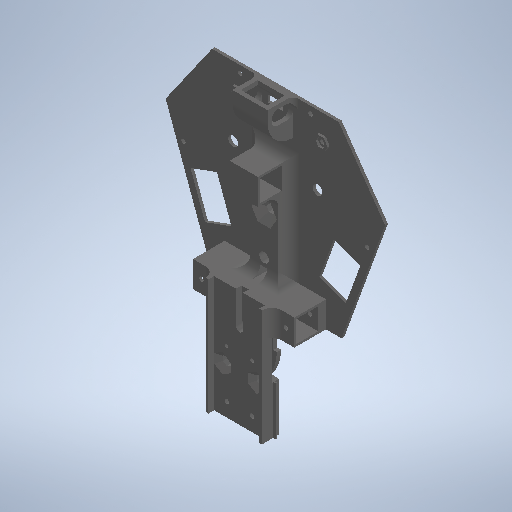
# Autodesk Inventor part: back_board_setter
Saved by Autodesk Inventor 2026.1 (Build 301233020, 233B)
## iProperties
Created: 2026-02-04
Part Number: back_board_setter
Material: 一般
Document SubType Name: Modeling
Designer: hibik
Density: 1 g/cm^3
Appearance: 既定
Author: hibik
Autodesk Inventor part; units mm, degrees
ref_plane "YZ Plane" through (0, 0, 0) normal (1, 0, 0) x (0, 1, 0)
ref_plane "XY Plane" through (0, 0, 0) normal (0, 0, 1) x (1, 0, 0)
sketch "スケッチ1" plane through (0, 0, 0) normal (0, 0, 1) x (1, 0, 0)
  line L0 (-36, -9.25) -> (36, -9.25)
  line L1 (36, -9.25) -> (36, 9.25)
  line L2 (36, 9.25) -> (-36, 9.25)
  line L3 (-36, 9.25) -> (-36, -9.25)
  point P0 (0, 0)
  point P1 (0, 9.25)
  point P2 (-36, 0)
  dimension "d0" = 72
  dimension "d1" = 18.5
  constraints: 8 end point, 2 midpoint, 2 parallel, 1 horizontal, 1 horizontal alignment, 1 perpendicular, 1 vertical alignment
  measures "d0" distance of L2.end L1.end
  measures "d1" distance of L2.end L0.start
extrude "押し出し1" add sketch "スケッチ1" along normal mid plane 18.5
shell "シェル1" thickness 1.5 removed faces 2 at (36, 3.0833, 3.0833) at (-36, 3.0833, -3.0833)
sketch "スケッチ2" plane through (0, 0, 9.25) normal (0, 0, 1) x (1, 0, 0)
  circle A0 centre (-30, 0) radius 1.6
  line L0 (0, -12.95) -> (0, 12.95) projected
  circle A1 centre (30, 0) radius 1.6
  line L1 (-36, 9.25) -> (-36, -9.25) projected
  point P0 (0, 0)
  dimension "d5" = 3.2
  dimension "d6" = 6
  constraints: 2 centre point, 1 horizontal alignment, 1 other
  measures "d5" diameter of A0
  measures "d6" distance from line of L1 A0.centre
extrude "押し出し2" cut sketch "スケッチ2" against normal through all
sketch "スケッチ3" plane through (0, 0, -9.25) normal (0, 0, -1) x (-1, 0, 0)
  line L0 (-10, 64.25) -> (10, 64.25)
  line L1 (10, 64.25) -> (10, -9.25)
  line L2 (10, -9.25) -> (-10, -9.25)
  line L3 (-10, -9.25) -> (-10, 64.25)
  line L4 (-36, -9.25) -> (36, -9.25) projected
  line L5 (-36, 9.25) -> (36, 9.25) projected
  line L6 (-10, 9.25) -> (10, 9.25)
  point P0 (0, 0)
  point P1 (0, -9.25)
  dimension "d14" = 64.25
  dimension "d15" = 20
  constraints: 10 end point, 4 point on line, 2 parallel, 1 collinear, 1 horizontal, 1 midpoint, 1 perpendicular, 1 vertical alignment
  measures "d14" distance from line of L0 point (0, 0)
  measures "d15" distance of L0.start L0.end
extrude "押し出し3" add sketch "スケッチ3" along normal mid plane 8 contours L0 L1 L5 L3
ref_plane "作業平面1" through (0, 73.5, 0) normal (0, 1, 0) x (-1, 0, 0)
sketch "スケッチ4" plane through (0, 0, 0) normal (1, 0, 0) x (0, 1, 0)
  line L0 (73.5, 14.95) -> (73.5, -24.95) projected
  line L1 (81.25, 7.75) -> (65.75, 7.75)
  line L2 (65.75, 7.75) -> (65.75, -7.75)
  line L3 (65.75, -7.75) -> (81.25, -7.75)
  line L4 (81.25, -7.75) -> (81.25, 7.75)
  line L5 (81.25, 7.75) -> (65.75, -7.75) construction
  line L6 (65.75, 7.75) -> (81.25, -7.75) construction
  line L7 (7.75, -7.75) -> (-7.75, -7.75) projected
  line L8 (82.75, 9.25) -> (64.25, 9.25)
  line L9 (64.25, 9.25) -> (64.25, -9.25)
  line L10 (64.25, -9.25) -> (82.75, -9.25)
  line L11 (82.75, -9.25) -> (82.75, 9.25)
  line L12 (82.75, 9.25) -> (64.25, -9.25) construction
  line L13 (64.25, 9.25) -> (82.75, -9.25) construction
  line L14 (-9.25, 9.25) -> (9.25, 9.25) projected
  point P0 (0, 0)
  point P1 (73.5, 0)
  constraints: 24 end point, 4 equal length, 4 midpoint, 4 parallel, 2 horizontal, 2 perpendicular, 1 horizontal alignment, 1 point on line
extrude "押し出し4" add sketch "スケッチ4" along normal mid plane 20 contours L8 L11 L10 L0 L3 L4 L1 | L0 L1 L2 L3 L10 L9 L8
sketch "スケッチ7" plane through (0, 0, 9.25) normal (0, 0, 1) x (1, 0, 0)
  line L0 (-36, 9.25) -> (-10, 9.25) projected
  line L1 (-20, 9.25) -> (20, 9.25)
  line L2 (20, 9.25) -> (20, -73.25)
  line L3 (20, -73.25) -> (-20, -73.25)
  line L4 (-20, -73.25) -> (-20, 9.25)
  line L5 (-36, -9.25) -> (36, -9.25) projected
  point P0 (0, 0)
  point P1 (0, -73.25)
  point P2 (-10, 9.25)
  dimension "d27" = 40
  dimension "d28" = 64
  constraints: 8 end point, 2 parallel, 1 horizontal, 1 midpoint, 1 perpendicular, 1 point on line, 1 vertical alignment
  measures "d27" distance of L2.end L3.end
  measures "d28" distance between parallel lines of L3 L5
extrude "押し出し7" add sketch "スケッチ7" along normal blind 7
sketch "スケッチ8" plane through (0, 0, 16.25) normal (0, 0, 1) x (1, 0, 0)
  line L0 (10, 9.25) -> (36, 9.25) projected
  line L1 (-18, -73.25) -> (18, -73.25)
  line L2 (18, -73.25) -> (18, 9.25)
  line L3 (18, 9.25) -> (-18, 9.25)
  line L4 (-18, 9.25) -> (-18, -73.25)
  line L5 (-20, -73.25) -> (20, -73.25) projected
  line L6 (-20, 9.25) -> (-20, -73.25) projected
  point P0 (0, 0)
  point P1 (0, -73.25)
  dimension "d31" = 2
  constraints: 8 end point, 2 midpoint, 2 parallel, 2 point on line, 1 horizontal, 1 perpendicular
  measures "d31" distance between parallel lines of L6 L4
extrude "押し出し8" cut sketch "スケッチ8" against normal blind 4
sketch "スケッチ9" plane through (0, 0, 9.25) normal (0, 0, -1) x (-1, 0, 0)
  line L0 (20, -9.25) -> (-20, -9.25) projected
  line L1 (-20, -73.25) -> (-20, -9.25) projected
  line L2 (20, -73.25) -> (-20, -73.25) projected
  line L3 (20, -9.25) -> (20, -73.25) projected
  point P0 (0, 0)
extrude "押し出し9" add sketch "スケッチ9" along normal blind 5
sketch "スケッチ10" plane through (0, 0, 4.25) normal (0, 0, -1) x (-1, 0, 0)
  circle A0 centre (-12, -41.25) radius 1.6
  line L0 (0, -104.45) -> (0, 113.95) projected
  circle A1 centre (12, -41.25) radius 1.6
  line L1 (-20, -9.25) -> (-20, -73.25) projected
  point P0 (0, 0)
  point P1 (-20, -41.25)
  dimension "d36" = 3.2
  dimension "d37" = 24
  constraints: 2 centre point, 1 horizontal alignment, 1 midpoint, 1 other
  measures "d36" diameter of A0
  measures "d37" distance of A1.centre A0.centre
extrude "押し出し10" cut sketch "スケッチ10" against normal through all
sketch "スケッチ11" plane through (0, 0, -13.25) normal (0, 0, -1) x (-1, 0, 0)
  line L0 (-72.5487, 98.7272) -> (-55.0126, 50.5473) projected
  line L1 (72.5487, 98.7272) -> (55.0126, 50.5473) projected
  line L2 (-95, 122.75) -> (95, 122.75)
  line L3 (95, 122.75) -> (46.9559, -9.25)
  line L4 (46.9559, -9.25) -> (-46.9559, -9.25)
  line L5 (-46.9559, -9.25) -> (-95, 122.75)
  line L6 (0, -107.6454) -> (0, 133.1226) projected
  line L7 (10, 82.75) -> (-10, 82.75) projected
  line L8 (-36, -9.25) -> (36, -9.25) projected
  point P0 (0, 0)
  dimension "d40" = 190
  dimension "d56" = 40
  constraints: 8 end point, 2 parallel, 1 collinear, 1 horizontal, 1 other
  measures "d40" distance of L2.start L2.end
  measures "d56" distance between parallel lines of L2 L7
extrude "押し出し11" add sketch "スケッチ11" along normal blind 2
sketch "スケッチ12" plane through (10, 82.75, -9.25) normal (0, 0, -1) x (-1, 0, 0)
  line L0 (20, 0) -> (0, 0) projected
  line L1 (0, -18.5) -> (0, 0) projected
  line L2 (20, -18.5) -> (0, -18.5) projected
  line L3 (20, 0) -> (20, -18.5) projected
  point P0 (10, -82.75)
extrude "押し出し12" add sketch "スケッチ12" along normal up to surface (4 mm away)
sketch "スケッチ13" plane through (0, 0, -9.25) normal (0, 0, -1) x (-1, 0, 0)
  circle A0 centre (-30, 0) radius 1.6 projected
  circle A1 centre (30, 0) radius 1.6 projected
  circle A2 centre (-30, 0) radius 3.5
  circle A3 centre (30, 0) radius 3.5
  circle A4 centre (30, 73.5) radius 1.6 projected
  circle A5 centre (-30, 73.5) radius 1.6 projected
  circle A6 centre (-30, 73.5) radius 3.5
  circle A7 centre (30, 73.5) radius 3.5
  point P0 (0, 0)
  dimension "d45" = 7
  dimension "d46" = 7
  dimension "d47" = 7
  dimension "d48" = 7
  constraints: 4 centre point, 4 coincident
  measures "d45" diameter of A2
  measures "d46" diameter of A3
  measures "d47" diameter of A6
  measures "d48" diameter of A7
extrude "押し出し13" cut sketch "スケッチ13" along normal through all contours A0 | A1 | A2 | A3 | A4 | A5 | A6 | A7
sketch "スケッチ14" plane through (0, 0, -15.25) normal (0, 0, -1) x (-1, 0, 0)
  circle A0 centre (30, 0) radius 3.5 projected
  line L0 (46.9559, -9.25) -> (95, 122.75) projected
  line L1 (95, 122.75) -> (-95, 122.75) projected
  line L2 (-95, 122.75) -> (-46.9559, -9.25) projected
  circle A1 centre (-30, 0) radius 3.5 projected
  line L3 (-46.9559, -9.25) -> (46.9559, -9.25) projected
  circle A2 centre (30, 73.5) radius 3.5 projected
  circle A3 centre (-30, 73.5) radius 3.5 projected
  circle A4 centre (30, 0) radius 1.6 projected
  circle A5 centre (-30, 0) radius 1.6 projected
  line L4 (-36, 9.25) -> (-36, -9.25) projected
  line L5 (-36, -9.25) -> (36, -9.25) projected
  line L6 (36, -9.25) -> (36, 9.25) projected
  line L7 (36, 9.25) -> (10, 9.25) projected
  line L8 (10, 9.25) -> (-10, 9.25) projected
  line L9 (-10, 9.25) -> (-36, 9.25) projected
  point P0 (0, 0)
  point P1 (33.2482, 9.25)
  point P2 (-33.2482, 9.25)
extrude "押し出し14" add sketch "スケッチ14" against normal up to surface (6 mm away) contours L3 L4 L9 L8 L7 L6
chamfer "面取り1" distance 50 angle 45 2 edges at (-95, 122.75, -14.25) (95, 122.75, -14.25)
fillet "フィレット3" radius 7 11 edges at (-10, 46, -13.25) (0, 82.75, -13.25) (10, 46, -13.25) (0, 9.25, -5.25) (-10, 9.25, -7.25) (-10, 9.25, -11.25) (10, 9.25, -11.25) (10, 9.25, -7.25) (-20, 0, 9.25) (20, 0, 9.25) (0, 64.25, -5.25)
sketch "スケッチ16" plane through (0, 0, -13.25) normal (0, 0, 1) x (1, 0, 0)
  line L0 (-60.2509, 41.8965) -> (-49.9903, 13.7058)
  line L1 (-49.9903, 13.7058) -> (-31.1964, 20.5462)
  line L2 (-31.1964, 20.5462) -> (-41.457, 48.7369)
  line L3 (-41.457, 48.7369) -> (-60.2509, 41.8965)
  line L4 (-46.9559, -9.25) -> (-77.899, 75.7654) projected
  point P0 (0, 0)
  point P1 (-43, 16.25)
  dimension "d66" = 5
  dimension "d67" = 20
  dimension "d68" = 30
  constraints: 8 end point, 3 parallel, 1 perpendicular, 1 point on line
  measures "d66" distance between parallel lines of L4 L0
  measures "d67" distance between parallel lines of L0 L2
  measures "d68" distance between parallel lines of L1 L3
extrude "押し出し16" cut sketch "スケッチ16" against normal through all
sketch "スケッチ17" plane through (0, 0, -13.25) normal (0, 0, 1) x (1, 0, 0)
  circle A0 centre (-65.2987, 55.7654) radius 1.6
  circle A1 centre (-65.2987, 55.7654) radius 5
  circle A2 centre (-25, 117.75) radius 5
  circle A3 centre (-25, 117.75) radius 1.6
  circle A4 centre (0, 21) radius 5
  circle A5 centre (0, 21) radius 1.6
  line L0 (-46.9559, -9.25) -> (-77.899, 75.7654) projected
  line L1 (-45, 122.75) -> (45, 122.75) projected
  point P0 (0, 0)
  dimension "d71" = 3.2
  dimension "d72" = 10
  dimension "d74" = 21
  dimension "d75" = 25
  dimension "d76" = 20
  constraints: 6 centre point, 4 equal radius, 3 coincident, 2 tangent, 1 vertical alignment
  measures "d71" diameter of A0
  measures "d72" diameter of A1
  measures "d74" distance of point (0, 0) A4.centre
  measures "d75" horizontal distance of point (0, 0) A2.centre
  measures "d76" vertical distance of L0.end A0.centre
extrude "押し出し17" cut sketch "スケッチ17" along normal mid plane 100 contours A0 | A3 | A5
sketch "スケッチ18" plane through (0, 0, -5.25) normal (0, 0, 1) x (1, 0, 0)
  circle A0 centre (0, 21) radius 1.6 projected
  circle A1 centre (0, 21) radius 3.5
  point P0 (0, 0)
  dimension "d79" = 7
  constraints: 1 centre point, 1 coincident
  measures "d79" diameter of A1
extrude "押し出し18" cut sketch "スケッチ18" against normal up to surface (8 mm away) contours A0 | A1
mirror "ミラー1" about plane through (0, 0, 0) normal (1, 0, 0) of "押し出し17", "押し出し16"
sketch "スケッチ19" plane through (-20, -9.25, 4.25) normal (0, -1, 0) x (1, 0, 0)
  line L0 (40, 12) -> (40, 0) projected
  line L1 (0, 0) -> (0, 12) projected
  line L2 (42, 3) -> (-2, 3)
  line L3 (-2, 3) -> (-2, 4)
  line L4 (-2, 4) -> (42, 4)
  line L5 (42, 4) -> (42, 3)
  line L6 (40, 0) -> (0, 0) projected
  point P0 (20, -4.25)
  point P1 (20, 0)
  point P2 (20, 3)
  point P3 (40, 4)
  point P4 (40, 3)
  point P5 (0, 3)
  point P6 (0, 4)
  dimension "d82" = 2
  dimension "d83" = 3
  dimension "d84" = 1
  constraints: 8 end point, 2 midpoint, 2 parallel, 1 horizontal, 1 perpendicular, 1 vertical alignment
  measures "d82" distance between parallel lines of L0 L5
  measures "d83" distance between parallel lines of L6 L2
  measures "d84" distance of L4.end L2.start
extrude "押し出し19" add sketch "スケッチ19" along normal up to surface (64 mm away) contours L4 L5 L2 L0 | L1 L2 L3 L4
sketch "スケッチ20" plane through (-45, 122.75, -13.25) normal (0, 1, 0) x (1, 0, 0)
  line L0 (54.5, -3) -> (35.5, -3)
  line L1 (35.5, -3) -> (35.5, -15)
  line L2 (35.5, -15) -> (54.5, -15)
  line L3 (54.5, -15) -> (54.5, -3)
  line L4 (57.5, 0) -> (32.5, 0)
  line L5 (32.5, 0) -> (32.5, -18)
  line L6 (32.5, -18) -> (57.5, -18)
  line L7 (57.5, -18) -> (57.5, 0)
  line L8 (0, 0) -> (90, 0) projected
  point P0 (45, -13.25)
  point P1 (54.5, -9)
  point P2 (57.5, -9)
  point P3 (45, 0)
  point P4 (45, 0)
  point P5 (45, -3)
  point P6 (45, 0)
  dimension "d87" = 19
  dimension "d88" = 12
  dimension "d89" = 3
  dimension "d90" = 3
  constraints: 16 end point, 6 midpoint, 4 parallel, 2 horizontal, 2 perpendicular, 1 coincident, 1 horizontal alignment, 1 point on line, 1 vertical alignment
  measures "d87" distance of L2.end L1.end
  measures "d88" distance of L1.end L0.end
  measures "d89" distance between parallel lines of L7 L3
  measures "d90" distance between parallel lines of L6 L2
extrude "押し出し20" add sketch "スケッチ20" against normal blind 3
sketch "スケッチ21" plane through (-12.5, 122.75, -13.25) normal (-1, 0, 0) x (0, 0, 1)
  line L0 (18, 0) -> (18, -3) projected
  line L1 (15, -3) -> (18, -3)
  line L2 (18, -3) -> (18, -8)
  line L3 (18, -8) -> (15, -8)
  line L4 (15, -8) -> (15, -3)
  arc A0 (0, -23) -> (15, -8) centre (0, -8) ccw
  arc A1 (0, -26) -> (18, -8) centre (0, -8) ccw
  line L5 (0, -3.4) -> (0, -6.6) projected
  line L6 (0, -65.3846) -> (0, -68.5846) projected
  line L7 (0, -65.3846) -> (0, -68.5846) projected
  line L8 (0, -3.4) -> (0, -6.6) projected
  line L9 (0, -45.75) -> (0, -52.75) projected
  line L10 (0, -45.75) -> (0, -52.75) projected
  line L11 (0, 0) -> (0, -3) projected
  line L12 (0, -3) -> (0, 0) projected
  line L13 (0, -46.9846) -> (0, 0) projected
  line L14 (0, -132) -> (0, -46.9846) projected
  line L15 (0, -102.2038) -> (0, -109.0442) projected
  line L16 (0, -109.0442) -> (0, -80.8535) projected
  line L17 (0, -80.8535) -> (0, -74.0131) projected
  line L18 (0, -74.0131) -> (0, -102.2038) projected
  line L19 (0, -33) -> (0, -113.5) projected
  line L20 (0, -113.5) -> (0, -33) projected
  line L21 (0, -109.0442) -> (0, -102.2038) projected
  line L22 (0, -102.2038) -> (0, -74.0131) projected
  line L23 (0, -74.0131) -> (0, -80.8535) projected
  line L24 (0, -80.8535) -> (0, -109.0442) projected
  line L25 (0, -46.9846) -> (0, -132) projected
  line L26 (0, 0) -> (0, -46.9846) projected
  line L27 (0, -23) -> (7.534, -23)
  line L28 (0, -132) -> (0, -113.5) projected
  line L29 (0, -113.5) -> (0, -132) projected
  point P0 (13.25, -122.75)
  point P1 (15, 0)
  point P2 (0, -23)
  dimension "d93" = 5
  constraints: 10 end point, 4 point on circle, 2 centre point, 2 horizontal, 2 parallel, 2 point on line, 2 tangent, 1 collinear, 1 concentric, 1 perpendicular
  measures "d93" distance of L1.end L2.end
extrude "押し出し21" add sketch "スケッチ21" against normal up to surface (25 mm away)
sketch "スケッチ22" plane through (0, 0, 4.25) normal (0, 0, -1) x (-1, 0, 0)
  line L0 (20, -9.25) -> (20, -73.25) projected
  line L1 (20, -19.25) -> (22.5, -19.25)
  arc A0 (16, -37.25) -> (22.5, -19.25) centre (-5.6731, -19.25) ccw
  line L2 (22.5, -19.25) -> (22.5, -28.0637)
  line L3 (16, -37.25) -> (16, -9.25)
  line L4 (16, -9.25) -> (20, -9.25)
  line L5 (-20, -9.25) -> (20, -9.25) projected
  line L6 (11.6828, -9.25) -> (37.771, -9.25)
  line L7 (37.771, -9.25) -> (37.771, -40.25)
  line L8 (37.771, -40.25) -> (11.6828, -40.25)
  line L9 (11.6828, -40.25) -> (11.6828, -9.25)
  circle A1 centre (20, -9.25) radius 29.6886
  point P0 (0, 0)
  point P1 (11.6828, -37.7498)
  point P2 (37.771, -33.0325)
  dimension "d96" = 4
  dimension "d97" = 2.5
  dimension "d98" = 10
  dimension "d99" = 18
  dimension "d100" = 3
  constraints: 16 end point, 3 perpendicular, 2 centre point, 2 horizontal, 2 parallel, 2 point on circle, 2 point on line, 1 coincident, 1 tangent, 1 vertical
  measures "d96" distance between parallel lines of L0 L3
  measures "d97" distance of L1.start L1.end
  measures "d98" distance from line of L1.start L4
  measures "d99" vertical distance of L1.end L3.start
  measures "d100" distance from line of L8 L3.start
extrude "押し出し22" cut sketch "スケッチ22" against normal blind 5 contours L6 L7 A1 L0 A0 L1 | L0 A0 L3 L4 | L1 A0 L0 | L3 A0 L0 A1 L9 L5
extrude "押し出し23" add sketch "スケッチ22" against normal blind 4 contours L0 A0 L3 L4 | L1 A0 L0
extrude "押し出し24" cut sketch "スケッチ22" against normal blind 1 contours L0 A0 L3 L4 | L1 A0 L0
mirror "ミラー2" about plane through (0, 0, 0) normal (1, 0, 0) of "押し出し22", "押し出し23", "押し出し24"
sketch "スケッチ23" plane through (0, 0, 12.25) normal (0, 0, 1) x (1, 0, 0)
  circle A0 centre (-9, -63.25) radius 1.3
  circle A1 centre (9, -63.25) radius 1.3
  line L0 (18, -73.25) -> (-18, -73.25) projected
  line L1 (0, -73.25) -> (0, 0)
  circle A2 centre (-9, -29.25) radius 1.3
  circle A3 centre (9, -29.25) radius 1.3
  dimension "d107" = 2.6
  dimension "d109" = 18
  dimension "d112" = 34
  dimension "d117" = 10
  constraints: 4 centre point, 2 end point, 2 vertical, 1 midpoint, 5 other
  measures "d107" diameter of A0
  measures "d109" distance of A1.centre A0.centre
  measures "d112" distance of A0.centre A2.centre
  measures "d117" distance from line of L0 A0.centre
extrude "押し出し25" cut sketch "スケッチ23" against normal up to surface (3 mm away)
sketch "スケッチ24" plane through (0, 0, 12.25) normal (0, 0, 1) x (1, 0, 0)
  circle A0 centre (-9, -63.25) radius 1.3 projected
  circle A1 centre (9, -63.25) radius 1.3 projected
  circle A2 centre (-9, -63.25) radius 1.6
  circle A3 centre (9, -63.25) radius 1.6
  point P0 (0, 0)
  dimension "d120" = 3.2
  dimension "d121" = 3.2
  constraints: 2 centre point, 2 coincident
  measures "d120" diameter of A2
  measures "d121" diameter of A3
extrude "押し出し26" cut sketch "スケッチ24" against normal through all contours A0 | A1 | A2 | A3
sketch "スケッチ25" plane through (0, 0, 4.25) normal (0, 0, -1) x (-1, 0, 0)
  circle A0 centre (-9, -63.25) radius 1.6 projected
  line L0 (-7.3546, -66.1) -> (-10.6454, -66.1)
  line L1 (-10.6454, -66.1) -> (-12.2909, -63.25)
  line L2 (-12.2909, -63.25) -> (-10.6454, -60.4)
  line L3 (-10.6454, -60.4) -> (-7.3546, -60.4)
  line L4 (-7.3546, -60.4) -> (-5.7091, -63.25)
  line L5 (-5.7091, -63.25) -> (-7.3546, -66.1)
  circle A1 centre (9, -63.25) radius 1.6 projected
  line L6 (7.3546, -66.1) -> (5.7091, -63.25)
  line L7 (5.7091, -63.25) -> (7.3546, -60.4)
  line L8 (7.3546, -60.4) -> (10.6454, -60.4)
  line L9 (10.6454, -60.4) -> (12.2909, -63.25)
  line L10 (12.2909, -63.25) -> (10.6454, -66.1)
  line L11 (10.6454, -66.1) -> (7.3546, -66.1)
  point P0 (0, 0)
  dimension "d124" = 5.7
  constraints: 24 end point, 2 coincident, 1 collinear, 1 horizontal, 1 horizontal alignment, 26 other
  measures "d124" distance between parallel lines of L0 L3
extrude "押し出し27" cut sketch "スケッチ25" against normal blind 6 contours A0 | L0 L1 L2 L3 L4 L5 | A1 | L6 L7 L8 L9 L10 L11
chamfer "面取り2" distance 4 angle 45 12 edges at (9, -60.4, 4.25) (6.5318, -61.825, 4.25) (6.5318, -64.675, 4.25) (9, -66.1, 4.25) (11.4682, -64.675, 4.25) (11.4682, -61.825, 4.25) (-6.5318, -61.825, 4.25) (-6.5318, -64.675, 4.25) (-9, -66.1, 4.25) (-11.4682, -64.675, 4.25) (-11.4682, -61.825, 4.25) (-9, -60.4, 4.25)
sketch "スケッチ26" plane through (0, 0, 12.25) normal (0, 0, 1) x (1, 0, 0)
  circle A0 centre (-12, -41.25) radius 1.6 projected
  circle A1 centre (12, -41.25) radius 1.6 projected
  line L0 (-9.15, -42.8954) -> (-12, -44.5409)
  line L1 (-12, -44.5409) -> (-14.85, -42.8954)
  line L2 (-14.85, -42.8954) -> (-14.85, -39.6046)
  line L3 (-14.85, -39.6046) -> (-12, -37.9591)
  line L4 (-12, -37.9591) -> (-9.15, -39.6046)
  line L5 (-9.15, -39.6046) -> (-9.15, -42.8954)
  line L6 (9.15, -42.8954) -> (9.15, -39.6046)
  line L7 (9.15, -39.6046) -> (12, -37.9591)
  line L8 (12, -37.9591) -> (14.85, -39.6046)
  line L9 (14.85, -39.6046) -> (14.85, -42.8954)
  line L10 (14.85, -42.8954) -> (12, -44.5409)
  line L11 (12, -44.5409) -> (9.15, -42.8954)
  point P0 (0, 0)
  dimension "d130" = 5.7
  dimension "d131" = 5.7
  constraints: 24 end point, 2 coincident, 2 vertical, 26 other
  measures "d130" distance between parallel lines of L5 L2
  measures "d131" distance from line of L9.end L6
extrude "押し出し28" cut sketch "スケッチ26" against normal blind 6 contours A0 | A1 | L0 L1 L2 L3 L4 L5 | L6 L7 L8 L9 L10 L11
chamfer "面取り3" distance 3 angle 45 12 edges at (-13.425, -43.7182, 12.25) (-14.85, -41.25, 12.25) (-13.425, -38.7818, 12.25) (-10.575, -38.7818, 12.25) (-9.15, -41.25, 12.25) (-10.575, -43.7182, 12.25) (9.15, -41.25, 12.25) (10.575, -38.7818, 12.25) (13.425, -38.7818, 12.25) (14.85, -41.25, 12.25) (13.425, -43.7182, 12.25) (10.575, -43.7182, 12.25)
sketch "スケッチ27" plane through (0, 0, -13.25) normal (0, 0, 1) x (1, 0, 0)
  line L0 (-12.5, 99.75) -> (12.5, 99.75) projected
  line L1 (-5.5, 99.75) -> (5.5, 99.75)
  line L2 (5.5, 99.75) -> (5.5, 114.75)
  line L3 (5.5, 114.75) -> (-5.5, 114.75)
  line L4 (-5.5, 114.75) -> (-5.5, 99.75)
  line L5 (-5.5, 109.75) -> (5.5, 109.75)
  point P0 (0, 0)
  point P1 (0, 99.75)
  dimension "d137" = 7
  dimension "d138" = 15
  dimension "d155" = 5
  constraints: 10 end point, 3 point on line, 2 midpoint, 2 parallel, 2 perpendicular, 1 horizontal
  measures "d137" distance from line of L4 L0.start
  measures "d138" distance of L3.end L1.start
  measures "d155" distance between parallel lines of L3 L5
extrude "押し出し29" cut sketch "スケッチ27" against normal through all contours L4 L3 L2 L5
sketch "スケッチ28" plane through (-12.5, 122.75, -13.25) normal (-1, 0, 0) x (0, 0, 1)
  arc A0 (0, -23) -> (15, -8) centre (0, -8) ccw projected
  line L0 (0, -13) -> (14.1421, -13)
  line L1 (0, -23) -> (0, -13)
  point P0 (13.25, -122.75)
  dimension "d141" = 10
  constraints: 4 end point, 1 perpendicular, 1 point on circle, 1 vertical
  measures "d141" distance of L1.start L0.start
extrude "押し出し30" add sketch "スケッチ28" against normal blind 3
mirror "ミラー3" about plane through (0, 0, 0) normal (1, 0, 0) of "押し出し30"
fillet "フィレット4" radius 4 9 edges at (0, 119.75, -13.25) (-11, 119.75, 1.75) (-11, 109.75, 0.8921) (-11, 109.75, -13.25) (-12.5, 121.25, -13.25) (12.5, 121.25, -13.25) (11, 109.75, -13.25) (11, 109.75, 0.8921) (11, 119.75, 1.75)
sketch "スケッチ29" plane through (0, 0, 0) normal (1, 0, 0) x (0, 1, 0)
  line L0 (9.25, -13.25) -> (9.25, 9.25) projected
  line L1 (-34.495, 12.25) -> (-37.8725, 12.25) projected
  line L2 (-37.8725, 12.25) -> (-34.495, 12.25) projected
  line L3 (-44.6275, 12.25) -> (-37.8725, 12.25) projected
  line L4 (-48.005, 12.25) -> (-44.6275, 12.25) projected
  line L5 (-44.6275, 12.25) -> (-48.005, 12.25) projected
  line L6 (-37.8725, 12.25) -> (-44.6275, 12.25) projected
  line L7 (-64.85, 12.25) -> (-61.65, 12.25) projected
  line L8 (-64.85, 12.25) -> (-61.65, 12.25) projected
  line L9 (-30.55, 12.25) -> (-27.95, 12.25) projected
  line L10 (-30.55, 12.25) -> (-27.95, 12.25) projected
  line L11 (9.25, 12.25) -> (-73.25, 12.25) projected
  line L12 (-73.25, 12.25) -> (9.25, 12.25) projected
  line L13 (-44.6275, 12.25) -> (-37.8725, 12.25) projected
  line L14 (-48.005, 12.25) -> (-44.6275, 12.25) projected
  line L15 (-44.6275, 12.25) -> (-48.005, 12.25) projected
  line L16 (-37.8725, 12.25) -> (-44.6275, 12.25) projected
  line L17 (-34.495, 12.25) -> (-37.8725, 12.25) projected
  line L18 (-37.8725, 12.25) -> (-34.495, 12.25) projected
  line L19 (9.25, 9.25) -> (9.25, 12.25)
  line L20 (9.25, 12.25) -> (15.25, 12.25)
  line L21 (15.25, 12.25) -> (15.25, -15.25)
  line L22 (15.25, -15.25) -> (9.25, -15.25)
  line L23 (9.25, -15.25) -> (9.25, 12.25)
  line L24 (-9.25, -15.25) -> (75.7654, -15.25) projected
  line L25 (9.25, 12.25) -> (-13.75, 12.25)
  line L26 (-13.75, 12.25) -> (-13.75, 8.25)
  line L27 (-13.75, 8.25) -> (9.25, 8.25)
  line L28 (9.25, 8.25) -> (9.25, 12.25)
  point P0 (0, 0)
  point P1 (-13.75, 12.25)
  dimension "d145" = 6
  dimension "d146" = 4
  dimension "d147" = 23
  constraints: 18 end point, 4 parallel, 2 horizontal, 2 perpendicular, 1 point on line, 1 vertical
  measures "d145" distance of L12.end L20.end
  measures "d146" distance between parallel lines of L12 L27
  measures "d147" distance of L26.end L27.end
extrude "押し出し31" cut sketch "スケッチ29" along normal mid plane 5
sketch "スケッチ30" plane through (0, 0, 12.25) normal (0, 0, 1) x (1, 0, 0)
  line L0 (2.5, -13.75) -> (-2.5, -13.75) projected
  circle A0 centre (0, -13.75) radius 2.5
  point P0 (0, 0)
  constraints: 1 horizontal alignment, 1 midpoint, 2 other
extrude "押し出し32" cut sketch "スケッチ30" against normal up to surface (8 mm away)
sketch "スケッチ32" plane through (0, 0, -15.25) normal (0, 0, -1) x (-1, 0, 0)
  circle A0 centre (-33.5, 104.75) radius 1.6 projected
  circle A1 centre (26.5, 104.75) radius 1.6 projected
  circle A2 centre (0, 48.75) radius 1.6 projected
  point P0 (0, 0)
extrude "押し出し33" cut sketch "スケッチ32" against normal through all
sketch "スケッチ33" plane through (0, 0, -13.25) normal (0, 0, 1) x (1, 0, 0)
  circle A0 centre (-26.5, 104.75) radius 1.6 projected
  circle A1 centre (33.5, 104.75) radius 1.6 projected
  line L0 (-24.8546, 101.9) -> (-28.1454, 101.9)
  line L1 (-28.1454, 101.9) -> (-29.7909, 104.75)
  line L2 (-29.7909, 104.75) -> (-28.1454, 107.6)
  line L3 (-28.1454, 107.6) -> (-24.8546, 107.6)
  line L4 (-24.8546, 107.6) -> (-23.2091, 104.75)
  line L5 (-23.2091, 104.75) -> (-24.8546, 101.9)
  line L6 (31.8546, 101.9) -> (30.2091, 104.75)
  line L7 (30.2091, 104.75) -> (31.8546, 107.6)
  line L8 (31.8546, 107.6) -> (35.1454, 107.6)
  line L9 (35.1454, 107.6) -> (36.7909, 104.75)
  line L10 (36.7909, 104.75) -> (35.1454, 101.9)
  line L11 (35.1454, 101.9) -> (31.8546, 101.9)
  line L12 (-23.9885, 109.1) -> (-21.4771, 104.75)
  line L13 (-21.4771, 104.75) -> (-23.9885, 100.4)
  line L14 (-23.9885, 100.4) -> (-29.0115, 100.4)
  line L15 (-29.0115, 100.4) -> (-31.5229, 104.75)
  line L16 (-31.5229, 104.75) -> (-29.0115, 109.1)
  line L17 (-29.0115, 109.1) -> (-23.9885, 109.1)
  line L18 (36.0115, 109.1) -> (38.5229, 104.75)
  line L19 (38.5229, 104.75) -> (36.0115, 100.4)
  line L20 (36.0115, 100.4) -> (30.9885, 100.4)
  line L21 (30.9885, 100.4) -> (28.4771, 104.75)
  line L22 (28.4771, 104.75) -> (30.9885, 109.1)
  line L23 (30.9885, 109.1) -> (36.0115, 109.1)
  point P0 (0, 0)
  point P1 (33.5, 107.6)
  dimension "d158" = 5.7
  dimension "d159" = 1.5
  constraints: 48 end point, 4 coincident, 3 horizontal, 2 collinear, 1 horizontal alignment, 1 midpoint, 52 other
  measures "d158" distance between parallel lines of L0 L3
  measures "d159" distance between parallel lines of L17 L3
extrude "押し出し34" add sketch "スケッチ33" along normal blind 1.5 contours L12 L13 L14 L15 L16 L17 | L18 L19 L20 L21 L22 L23
sketch "スケッチ34" plane through (0, 0, -5.25) normal (0, 0, 1) x (1, 0, 0)
  circle A0 centre (0, 48.75) radius 1.6 projected
  line L0 (1.6454, 45.9) -> (-1.6454, 45.9)
  line L1 (-1.6454, 45.9) -> (-3.2909, 48.75)
  line L2 (-3.2909, 48.75) -> (-1.6454, 51.6)
  line L3 (-1.6454, 51.6) -> (1.6454, 51.6)
  line L4 (1.6454, 51.6) -> (3.2909, 48.75)
  line L5 (3.2909, 48.75) -> (1.6454, 45.9)
  point P0 (0, 0)
  dimension "d162" = 5.7
  constraints: 12 end point, 1 coincident, 1 horizontal, 13 other
  measures "d162" distance between parallel lines of L0 L3
extrude "押し出し35" cut sketch "スケッチ34" against normal blind 8 contours A0 | L0 L1 L2 L3 L4 L5
chamfer "面取り4" distance 5 angle 45 6 edges at (0, 51.6, -5.25) (2.4682, 50.175, -5.25) (2.4682, 47.325, -5.25) (0, 45.9, -5.25) (-2.4682, 47.325, -5.25) (-2.4682, 50.175, -5.25)
equation "\"d131\" = d130"
